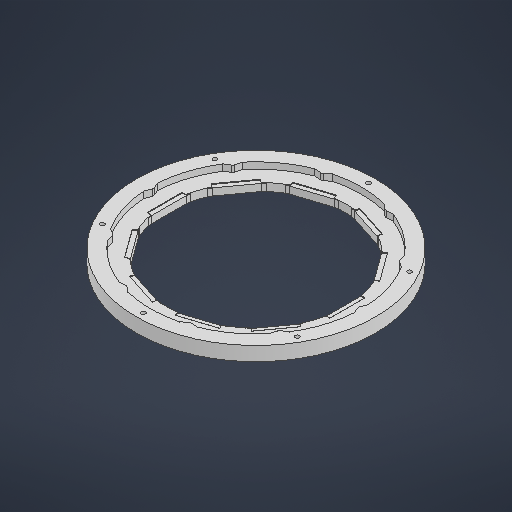
# Autodesk Inventor part: shell_base
Saved by Autodesk Inventor 2025 (Build 290162010, 162A)
## iProperties
Created: 2024-11-09
Part Number: shell_base
Material: Generic
Document SubType Name: Modeling
Designer: river
Density: 1 g/cm^3
Appearance: Default
Author: river
Autodesk Inventor part; units mm, degrees
ref_plane "YZ Plane" through (0, 0, 0) normal (1, 0, 0) x (0, 1, 0)
ref_plane "XZ Plane" through (0, 0, 0) normal (0, 1, 0) x (-1, 0, 0)
ref_plane "XY Plane" through (0, 0, 0) normal (0, 0, 1) x (1, 0, 0)
derived "lamina_rotor.ipt"
sketch "Sketch1" plane through (0, 0, 0) normal (0, 1, 0) x (-1, 0, 0)
  circle A0 centre (0, 0) radius 75
  circle A1 centre (0, 0) radius 63.5
  line L0 (62, 12.5) -> (62, -12.5)
  line L1 (62, -12.5) -> (65, -12.5)
  line L2 (65, -12.5) -> (65, 12.5)
  line L3 (65, 12.5) -> (62, 12.5)
  line L4 (62, 12.5) -> (65, -12.5) construction
  line L5 (62, -12.5) -> (65, 12.5) construction
  line L6 (75, 0) -> (0, 0) construction
  line L7 (59.9334, 28.0933) -> (45.2388, 48.3188)
  line L8 (45.2388, 48.3188) -> (42.8117, 46.5554)
  line L9 (42.8117, 46.5554) -> (57.5064, 26.33)
  line L10 (57.5064, 26.33) -> (59.9334, 28.0933)
  line L11 (31.9743, 57.956) -> (8.1979, 65.6814)
  line L12 (8.1979, 65.6814) -> (7.2708, 62.8282)
  line L13 (7.2708, 62.8282) -> (31.0473, 55.1028)
  line L14 (31.0473, 55.1028) -> (31.9743, 57.956)
  line L15 (-8.1979, 65.6814) -> (-31.9743, 57.956)
  line L16 (-31.9743, 57.956) -> (-31.0473, 55.1028)
  line L17 (-31.0473, 55.1028) -> (-7.2708, 62.8282)
  line L18 (-7.2708, 62.8282) -> (-8.1979, 65.6814)
  line L19 (-45.2388, 48.3188) -> (-59.9334, 28.0933)
  line L20 (-59.9334, 28.0933) -> (-57.5064, 26.33)
  line L21 (-57.5064, 26.33) -> (-42.8117, 46.5554)
  line L22 (-42.8117, 46.5554) -> (-45.2388, 48.3188)
  line L23 (-65, 12.5) -> (-65, -12.5)
  line L24 (-65, -12.5) -> (-62, -12.5)
  line L25 (-62, -12.5) -> (-62, 12.5)
  line L26 (-62, 12.5) -> (-65, 12.5)
  line L27 (-59.9334, -28.0933) -> (-45.2388, -48.3188)
  line L28 (-45.2388, -48.3188) -> (-42.8117, -46.5554)
  line L29 (-42.8117, -46.5554) -> (-57.5064, -26.33)
  line L30 (-57.5064, -26.33) -> (-59.9334, -28.0933)
  line L31 (-31.9743, -57.956) -> (-8.1979, -65.6814)
  line L32 (-8.1979, -65.6814) -> (-7.2708, -62.8282)
  line L33 (-7.2708, -62.8282) -> (-31.0473, -55.1028)
  line L34 (-31.0473, -55.1028) -> (-31.9743, -57.956)
  line L35 (8.1979, -65.6814) -> (31.9743, -57.956)
  line L36 (31.9743, -57.956) -> (31.0473, -55.1028)
  line L37 (31.0473, -55.1028) -> (7.2708, -62.8282)
  line L38 (7.2708, -62.8282) -> (8.1979, -65.6814)
  line L39 (45.2388, -48.3188) -> (59.9334, -28.0933)
  line L40 (59.9334, -28.0933) -> (57.5064, -26.33)
  line L41 (57.5064, -26.33) -> (42.8117, -46.5554)
  line L42 (42.8117, -46.5554) -> (45.2388, -48.3188)
  circle A2 centre (75, 0) radius 2
  line L43 (74.8331, 5) -> (73.1411, 0.738)
  line L44 (73.1411, -0.738) -> (74.8331, -5)
  circle A3 centre (60.6763, 44.0839) radius 2
  line L45 (57.6024, 48.0309) -> (58.7386, 43.5883)
  line L46 (59.6062, 42.3942) -> (63.4802, 39.9407)
  circle A4 centre (23.1763, 71.3292) radius 2
  line L47 (18.3694, 72.7156) -> (21.9, 69.7894)
  line L48 (23.3037, 69.3333) -> (27.88, 69.6255)
  circle A5 centre (-23.1763, 71.3292) radius 2
  line L49 (-27.88, 69.6255) -> (-23.3037, 69.3333)
  line L50 (-21.9, 69.7894) -> (-18.3694, 72.7156)
  circle A6 centre (-60.6763, 44.0839) radius 2
  line L51 (-63.4802, 39.9407) -> (-59.6062, 42.3942)
  line L52 (-58.7386, 43.5883) -> (-57.6024, 48.0309)
  circle A7 centre (-75, 0) radius 2
  line L53 (-74.8331, -5) -> (-73.1411, -0.738)
  line L54 (-73.1411, 0.738) -> (-74.8331, 5)
  circle A8 centre (-60.6763, -44.0839) radius 2
  line L55 (-57.6024, -48.0309) -> (-58.7386, -43.5883)
  line L56 (-59.6062, -42.3942) -> (-63.4802, -39.9407)
  circle A9 centre (-23.1763, -71.3292) radius 2
  line L57 (-18.3694, -72.7156) -> (-21.9, -69.7894)
  line L58 (-23.3037, -69.3333) -> (-27.88, -69.6255)
  circle A10 centre (23.1763, -71.3292) radius 2
  line L59 (27.88, -69.6255) -> (23.3037, -69.3333)
  line L60 (21.9, -69.7894) -> (18.3694, -72.7156)
  circle A11 centre (60.6763, -44.0839) radius 2
  line L61 (63.4802, -39.9407) -> (59.6062, -42.3942)
  line L62 (58.7386, -43.5883) -> (57.6024, -48.0309)
  circle A12 centre (0, 0) radius 85
  circle A13 centre (0, -80) radius 1.5
  line L63 (0, -80) -> (0, -75) construction
  circle A14 centre (69.282, -40) radius 1.5
  circle A15 centre (69.282, 40) radius 1.5
  circle A16 centre (0, 80) radius 1.5
  circle A17 centre (-69.282, 40) radius 1.5
  circle A18 centre (-69.282, -40) radius 1.5
  line L64 (62, -12.5) -> (61.6972, -15.0237)
  line L65 (62, 12.5) -> (61.6972, 15.0237)
  line L66 (42.8117, 46.5554) -> (41.0834, 48.4191)
  line L67 (57.5064, 26.33) -> (58.7447, 24.1103)
  line L68 (7.2708, 62.8282) -> (4.7771, 63.3201)
  line L69 (31.0473, 55.1028) -> (33.3538, 54.0349)
  line L70 (-31.0473, 55.1028) -> (-33.3538, 54.0349)
  line L71 (-7.2708, 62.8282) -> (-4.7771, 63.3201)
  line L72 (-57.5064, 26.33) -> (-58.7447, 24.1103)
  line L73 (-42.8117, 46.5554) -> (-41.0834, 48.4191)
  line L74 (-62, -12.5) -> (-61.6972, -15.0237)
  line L75 (-62, 12.5) -> (-61.6972, 15.0237)
  line L76 (-42.8117, -46.5554) -> (-41.0834, -48.4191)
  line L77 (-57.5064, -26.33) -> (-58.7447, -24.1103)
  line L78 (-7.2708, -62.8282) -> (-4.7771, -63.3201)
  line L79 (-31.0473, -55.1028) -> (-33.3538, -54.0349)
  line L80 (31.0473, -55.1028) -> (33.3538, -54.0349)
  line L81 (7.2708, -62.8282) -> (4.7771, -63.3201)
  line L82 (57.5064, -26.33) -> (58.7447, -24.1103)
  line L83 (42.8117, -46.5554) -> (41.0834, -48.4191)
  point P0 (63.5, 0)
  point P1 (63.5, 0)
  point P2 (65, 0)
  point P3 (43.0201, -46.7068)
  point P4 (31.1268, -55.3477)
  point P5 (7.3504, -63.0731)
  point P6 (-7.3504, -63.0731)
  point P7 (-31.1268, -55.3477)
  point P8 (-43.0201, -46.7068)
  point P9 (-57.7147, -26.4813)
  point P10 (-62.2575, -12.5)
  point P11 (-62.2575, 12.5)
  point P12 (-57.7147, 26.4813)
  point P13 (-43.0201, 46.7068)
  point P14 (-31.1268, 55.3477)
  point P15 (-7.3504, 63.0731)
  point P16 (7.3504, 63.0731)
  point P17 (31.1268, 55.3477)
  point P18 (43.0201, 46.7068)
  point P19 (57.7147, 26.4813)
  point P20 (62.2575, 12.5)
  point P21 (62.2575, -12.5)
  point P22 (57.7147, -26.4813)
  dimension "d1" = 170
  dimension "d2" = 3
  dimension "d3" = 5
  dimension "d6" = 360
  dimension "d16" = 360
  measures "d1" diameter of A12
  measures "d2" diameter of A13
  measures "d3" distance of L63.start L63.end
extrude "Extrusion1" add sketch "Sketch1" against normal blind 10 contours L43 A2 L44 A0 L61 A11 L62 L59 A10 L60 L57 A9 L58 L55 A8 L56 L53 A7 L54 L51 A6 L52 L49 A5 L50 L47 A4 L48 L45 A3 L46 | A0 A2 L43 | L46 A3 A0 | A2 A0 | A0 A2 | A3 A0 | A0 A3 | A2 A0 L44 | A3 L45 A0 | A0 A11 L61 | L48 A4 A0 | A11 A0 | A0 A11 | A4 A0 | A0 A4 | A0 L62 A11 | A4 L47 A0 | A0 A10 L59 | L50 A5 A0 | A10 A0 | A0 A10 | A5 A0 | A0 A5 | A0 L60 A10 | A5 L49 A0 | A0 A9 L57 | L52 A6 A0 | A9 A0 | A0 A9 | A6 A0 | A0 A6 | A0 L58 A9 | A6 L51 A0 | A0 A8 L55 | L54 A7 A0 | A8 A0 | A0 A8 | A7 A0 | A0 A7 | A0 L56 A8 | A7 L53 A0 | A1 L3 L65 | L67 L10 A1 | L3 L2 L1 A1 | A1 L1 L0 L3 | L10 L9 L8 A1 | A1 L8 L7 L10 | L1 A1 L64 | L8 L66 A1 | A1 L40 L82 | L69 L14 A1 | L40 L39 L42 A1 | A1 L42 L41 L40 | L14 L13 L12 A1 | A1 L12 L11 L14 | A1 L83 L42 | L12 L68 A1 | A1 L36 L80 | L71 L18 A1 | L36 L35 L38 A1 | A1 L38 L37 L36 | L18 L17 L16 A1 | A1 L16 L15 L18 | A1 L81 L38 | L16 L70 A1 | A1 L32 L78 | L73 L22 A1 | L32 L31 L34 A1 | A1 L34 L33 L32 | L22 L21 L20 A1 | A1 L20 L19 L22 | A1 L79 L34 | L20 L72 A1 | A1 L28 L76 | L75 L26 A1 | L28 L27 L30 A1 | A1 L30 L29 L28 | L26 L25 L24 A1 | A1 L24 L23 L26 | A1 L77 L30 | L24 L74 A1 | A12
extrude "Extrusion2" cut sketch "Sketch1" against normal blind 4.5 contours L43 A2 L44 A0 L61 A11 L62 L59 A10 L60 L57 A9 L58 L55 A8 L56 L53 A7 L54 L51 A6 L52 L49 A5 L50 L47 A4 L48 L45 A3 L46
extrude "Extrusion3" cut sketch "Sketch1" against normal blind 5 contours A1 L3 L65 | L67 L10 A1 | L3 L2 L1 A1 | A1 L1 L0 L3 | L10 L9 L8 A1 | A1 L8 L7 L10 | L1 A1 L64 | L8 L66 A1 | A1 L40 L82 | L69 L14 A1 | L40 L39 L42 A1 | A1 L42 L41 L40 | L14 L13 L12 A1 | A1 L12 L11 L14 | A1 L83 L42 | L12 L68 A1 | A1 L36 L80 | L71 L18 A1 | L36 L35 L38 A1 | A1 L38 L37 L36 | L18 L17 L16 A1 | A1 L16 L15 L18 | A1 L81 L38 | L16 L70 A1 | A1 L32 L78 | L73 L22 A1 | L32 L31 L34 A1 | A1 L34 L33 L32 | L22 L21 L20 A1 | A1 L20 L19 L22 | A1 L79 L34 | L20 L72 A1 | A1 L28 L76 | L75 L26 A1 | L28 L27 L30 A1 | A1 L30 L29 L28 | L26 L25 L24 A1 | A1 L24 L23 L26 | A1 L77 L30 | L24 L74 A1
body "Solid2"
